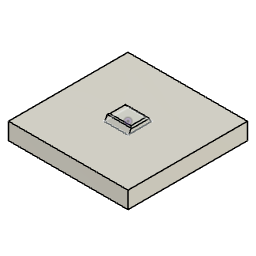
AU_switch (Autodesk Fusion 360 design; units mm, degrees)
Autodesk Fusion 360 part; units mm, degrees
note: some values were not read from the file. Set by a fixed rule: which sketch regions a step uses.
box "BoxPrimitive3" add length 85 width 85 height 12 placed x (0, 1, 0) y (-1, 0, 0) z (0, 0, 1) at (85, 0, 0) makes body 1 in component "panel"
sketch "Sketch1" plane through (0, 0, 0) normal (0, 1, 0) x (1, 0, 0) in component "button"
  line L0 (52, -32) -> (40, -32)
  line L1 (40, -32) -> (37.0938, -26.1859)
  line L2 (52, -32) -> (54.9063, -26.1859)
  line L3 (52, -32) -> (40, -32) construction
  line L4 (40, -20.3718) -> (37.0938, -26.1859)
  line L5 (52, -20.3718) -> (40, -20.3718)
  line L6 (52, -20.3718) -> (54.9063, -26.1859)
  line L7 (38.5469, -29.093) -> (46, -25.3674) construction
  line L8 (46, -32) -> (46, -25.3674) construction
  line L9 (53.4531, -29.093) -> (46, -25.3674) construction
  line L10 (37.0938, -26.1859) -> (52, -32) construction
  point P0 (46, -25.3674)
  dimension "d32" = 12
  dimension "d33" = 16
  dimension "d34" = 16
  dimension "d50" = 6.5
  dimension "d51" = 6.5
  constraint horizontal L0
  constraint horizontal L3
  constraint equal L0 L5
  constraint equal L2 L4
  constraint equal L1 L6
  constraint midpoint L1 L7.start
  constraint perpendicular L1 L7
  constraint midpoint L3 L8.start
  constraint perpendicular L0 L8
  constraint midpoint L2 L9.start
  constraint perpendicular L2 L9
  constraint coincident L8 P0
  constraint coincident L7 P0
  constraint coincident P0 L7.end
  measures "d32" distance of L0.start L0.end
  measures "d33" distance of L0.end L2.end
  measures "d34" distance of L0.start L1.end
  measures "d50" distance of L0.end L1.end
  measures "d51" distance of L0.start L2.end
extrude "Extrude1" add sketch "Sketch1" along normal blind 17 separate body makes body 2 in component "button"
fillet "Fillet1" radius 2 2 edges at (37.0938, 8.5, 26.1859) (54.9063, 8.5, 26.1859) on bodies 2 in component "button"
fillet "Fillet1" radius 1 2 faces at (48, 11.3333, 32) (48, 11.3333, 20.3718) on bodies 2 in component "button"
ref_plane "WorkPlane1" through (46, 8.5, 26.1859) normal (0, 1, 0) x (0, 0, 1) in component "button"
ref_plane "WorkPlane1" through (42.5, 42.5, 12) normal (0, 0, 1) x (0, 1, 0) in component "panel"
sketch "Sketch5" plane through (42.5, 42.5, 12) normal (0, 0, 1) x (1, 0, 0) in component "panel"
  line L0 (-8.5, 8.5) -> (8.5, 8.5)
  line L1 (8.5, 8.5) -> (8.5, -8.5)
  line L2 (8.5, -8.5) -> (-8.5, -8.5)
  line L3 (-8.5, -8.5) -> (-8.5, 8.5)
  dimension "d59" = 17
  dimension "d60" = 17
  dimension "d61" = 8.5
  dimension "d63" = 8.5
  constraint horizontal L0
  constraint vertical L1
  constraint horizontal L2
  constraint vertical L3
  measures "d59" distance of L0.start L0.end
  measures "d60" distance of L0.start L2.end
  measures "d61" distance of origin L1
  measures "d63" distance of origin L0
extrude "Extrude3" cut sketch "Sketch5" against normal through all bodies 1 in component "panel"
ref_plane "WorkPlane2" through (42.5, 42.5, 0) normal (0, 0, -1) x (0, -1, 0) in component "panel"
sketch "Sketch7" plane through (42.5, 42.5, 0) normal (0, 0, -1) x (1, 0, 0) in component "panel"
  line L0 (-40, 40) -> (40, 40)
  line L1 (40, 40) -> (40, -40)
  line L2 (40, -40) -> (-40, -40)
  line L3 (-40, -40) -> (-40, 40)
  line L4 (-8.5, 13) -> (8.5, 13)
  line L5 (8.5, 13) -> (8.5, -13)
  line L6 (8.5, -13) -> (-8.5, -13)
  line L7 (-8.5, -13) -> (-8.5, 13)
  dimension "d66" = 26
  dimension "d67" = 17
  dimension "d68" = 8.5
  dimension "d69" = 13
  dimension "d70" = 40
  dimension "d71" = 80
  dimension "d72" = 80
  dimension "d73" = 40
  constraint horizontal L0
  constraint vertical L1
  constraint horizontal L2
  constraint vertical L3
  constraint horizontal L4
  constraint vertical L5
  constraint horizontal L6
  constraint vertical L7
  measures "d66" distance of L4.start L6.end
  measures "d67" distance of L4.start L4.end
  measures "d68" distance of origin L5
  measures "d69" distance of origin L4
  measures "d70" distance of origin L1
  measures "d71" distance of L1.end L2.end
  measures "d72" distance of L0.start L2.end
  measures "d73" distance of origin L2
extrude "Extrude4" cut sketch "Sketch7" against normal blind 10 bodies 1 in component "panel"
ref_plane "WorkPlane3" through (42.5, 42.5, 6) normal (0, -1, 0) x (-1, 0, 0) in component "panel"
sketch "Sketch8" plane through (42.5, 42.5, 6) normal (0, -1, 0) x (1, 0, 0) in component "panel"
  circle A0 centre (0.0246, 2.001) radius 1.5
  line L0 (8.5, 6) -> (-8.5, 6)
  dimension "d76" = 3
  dimension "d87" = 3.999
  measures "d76" diameter of A0
  measures "d87" distance of A0.centre L0
extrude "Extrude5" cut sketch "Sketch8" along normal mid plane 26 bodies 1 in component "panel"
sketch "Sketch3" plane through (46, 8.5, 26.1859) normal (0, 1, 0) x (1, 0, 0) in component "button"
  circle A0 centre (0, 1.8189) radius 1.5
  line L0 (-6.4999, -4.8141) -> (6.4999, -4.8141)
  dimension "d79" = 3
  dimension "d86" = 6.633
  measures "d79" diameter of A0
  measures "d86" distance of A0.centre L0
extrude "Extrude3'" add sketch "Sketch3" along normal mid plane 26 bodies 2 in component "button"
fillet "Fillet2" radius 2 2 edges at (34, 42.5, 10) (51, 42.5, 10) on bodies 1 in component "panel"
component "panel" placed x (1, 0, 0) y (0, 1, 0) z (0, 0, 1) at (0, 0, 0)
component "button" placed x (1, 0, 0) y (0, 1, 0) z (0, 0, 1) at (-3.4754, 34, -16.366)
named bodies: "Body1"
